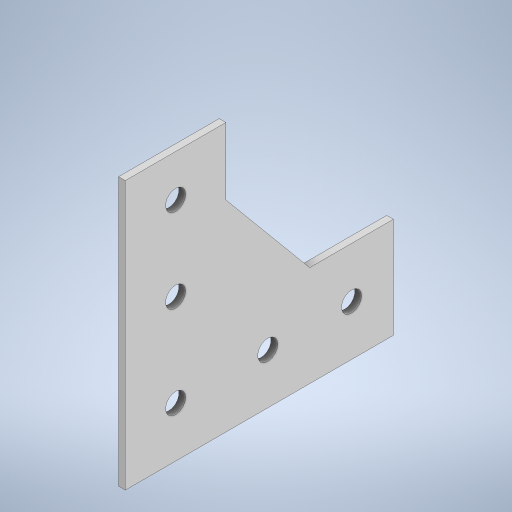
# Autodesk Inventor part: Connect2x3030_m6
Saved by Autodesk Inventor 2024 (Build 280153000, 153)
## iProperties
Created: 2025-12-08
Part Number: Connect2x3030_m6
Material: Generic
Document SubType Name: Modeling
Designer: schar
Density: 1 g/cm^3
Appearance: Default
Author: schar
Autodesk Inventor part; units mm, degrees
ref_plane "YZ Plane" through (0, 0, 0) normal (1, 0, 0) x (0, 1, 0)
ref_plane "XZ Plane" through (0, 0, 0) normal (0, 1, 0) x (-1, 0, 0)
ref_plane "XY Plane" through (0, 0, 0) normal (0, 0, 1) x (1, 0, 0)
sketch "Sketch4" plane through (0, 0, 0) normal (1, 0, 0) x (0, 1, 0)
  line L0 (0, 0) -> (80, 0)
  line L1 (80, 0) -> (80, -30)
  line L2 (80, -30) -> (0, -30)
  line L3 (0, -30) -> (0, 0)
  line L4 (0, -30) -> (30, -30)
  line L5 (30, -30) -> (30, -80)
  line L6 (30, -80) -> (0, -80)
  line L7 (0, -80) -> (0, -30)
  line L8 (80, -30) -> (60, -30)
  line L9 (60, -30) -> (30, -55)
  dimension "d10" = 80
  dimension "d11" = 30
  dimension "d12" = 30
  dimension "d13" = 50
  dimension "d14" = 20
  constraints: 20 end point, 4 parallel, 2 horizontal, 2 perpendicular, 1 midpoint, 1 point on line
  measures "d10" distance of L1.end L2.end
  measures "d11" distance of L0.end L1.end
  measures "d12" distance of L5.end L6.end
  measures "d13" distance of L4.end L5.end
  measures "d14" distance of L1.end L8.end
extrude "Extrusion2" add sketch "Sketch4" along normal blind 2
sketch "Sketch6" plane through (2, 0, 0) normal (1, 0, 0) x (0, 0, -1)
  line L0 (0, 0) -> (80, 0) projected
  line L1 (80, 0) -> (80, 15)
  line L2 (80, 0) -> (80, 30) projected
  line L3 (80, 15) -> (67.5, 15)
  line L4 (80, 15) -> (30, 15)
  line L5 (30, 15) -> (42.5, 15)
  line L6 (0, 0) -> (15, 0)
  line L7 (15, 0) -> (15, 15)
  line L8 (30, 80) -> (0, 80) projected
  line L9 (0, 80) -> (15, 80)
  line L10 (15, 80) -> (15, 30)
  line L11 (15, 30) -> (15, 42.5)
  line L12 (15, 80) -> (15, 67.5)
  dimension "d47" = 12.5
  dimension "d48" = 50
  dimension "d49" = 12.5
  dimension "d50" = 15
  dimension "d51" = 15
  dimension "d52" = 15
  dimension "d53" = 50
  dimension "d54" = 12.5
  dimension "d55" = 12.5
  constraints: 20 end point, 4 point on line, 3 perpendicular, 2 midpoint, 1 horizontal
  measures "d47" distance of L1.end L3.end
  measures "d48" distance of L1.end L4.end
  measures "d49" distance of L4.end L5.end
  measures "d50" distance of L0.start L6.end
  measures "d51" distance of L6.end L7.end
  measures "d52" distance of L8.end L9.end
  measures "d53" distance of L9.end L10.end
  measures "d54" distance of L10.end L11.end
  measures "d55" distance of L9.end L12.end
hole "Hole2" at (2, 67.5, -15) at (2, 42.5, -15) at (2, 15, -15) at (2, 15, -42.5) at (2, 15, -67.5) direction (-1, 0, 0) diameter 6 end through all
body "Solid2"
